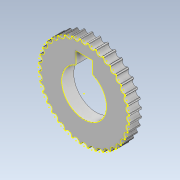
# Autodesk Inventor part: 2GT_36T
Saved by Autodesk Inventor 2022 (Build 260153000, 153)
## iProperties
Created: 2023-05-04
Part Number: 2GT_36T
Material: 一般
Document SubType Name: Modeling
Designer: Johnny Jou
Density: 1 g/cm^3
Appearance: 預設
Author: Johnny Jou
Autodesk Inventor part; units mm, degrees
ref_plane "YZ Plane" through (0, 0, 0) normal (1, 0, 0) x (0, 1, 0)
ref_plane "XZ Plane" through (0, 0, 0) normal (0, 1, 0) x (-1, 0, 0)
ref_plane "XY Plane" through (0, 0, 0) normal (0, 0, 1) x (1, 0, 0)
sketch "草圖1" plane through (0, 0, 0) normal (0, 0, 1) x (1, 0, 0)
  arc A0 (-2.6557, 10.7931) -> (-2.7562, 10.8607) centre (-2.7504, 10.7609) ccw
  arc A1 (-2.7562, 10.8607) -> (-3.0435, 10.7838) centre (0, 0) ccw
  arc A2 (-3.0435, 10.7838) -> (-3.0966, 10.675) centre (-2.9985, 10.6944) ccw
  arc A3 (-4.4896, 10.168) -> (-3.0966, 10.675) centre (-3.8323, 10.5293) ccw
  arc A4 (-4.4896, 10.168) -> (-4.6002, 10.2171) centre (-4.5772, 10.1198) ccw
  arc A5 (-4.6002, 10.2171) -> (-4.8698, 10.0914) centre (0, 0) ccw
  arc A6 (-4.8698, 10.0914) -> (-4.9033, 9.9751) centre (-4.81, 10.0113) ccw
  arc A7 (-6.187, 9.2339) -> (-4.9033, 9.9751) centre (-5.6025, 9.7038) ccw
  arc A8 (-6.187, 9.2339) -> (-6.3045, 9.2631) centre (-6.265, 9.1713) ccw
  arc A9 (-6.3045, 9.2631) -> (-6.5482, 9.0925) centre (0, 0) ccw
  arc A10 (-6.5482, 9.0925) -> (-6.5609, 8.9721) centre (-6.4754, 9.0239) ccw
  arc A11 (-7.6965, 8.0193) -> (-6.5609, 8.9721) centre (-7.2024, 8.5835) ccw
  arc A12 (-7.6965, 8.0193) -> (-7.8173, 8.0276) centre (-7.7624, 7.944) ccw
  arc A13 (-7.8173, 8.0276) -> (-8.0276, 7.8173) centre (0, 0) ccw
  arc A14 (-8.0276, 7.8173) -> (-8.0193, 7.6965) centre (-7.944, 7.7624) ccw
  arc A15 (-8.9721, 6.5609) -> (-8.0193, 7.6965) centre (-8.5835, 7.2024) ccw
  arc A16 (-8.9721, 6.5609) -> (-9.0925, 6.5482) centre (-9.0239, 6.4754) ccw
  arc A17 (-9.0925, 6.5482) -> (-9.2631, 6.3045) centre (0, 0) ccw
  arc A18 (-9.2631, 6.3045) -> (-9.2339, 6.187) centre (-9.1713, 6.265) ccw
  arc A19 (-9.9751, 4.9033) -> (-9.2339, 6.187) centre (-9.7038, 5.6025) ccw
  arc A20 (-9.9751, 4.9033) -> (-10.0914, 4.8698) centre (-10.0113, 4.81) ccw
  arc A21 (-10.0914, 4.8698) -> (-10.2171, 4.6002) centre (0, 0) ccw
  arc A22 (-10.2171, 4.6002) -> (-10.168, 4.4896) centre (-10.1198, 4.5772) ccw
  arc A23 (-10.675, 3.0966) -> (-10.168, 4.4896) centre (-10.5293, 3.8323) ccw
  arc A24 (-10.675, 3.0966) -> (-10.7838, 3.0435) centre (-10.6944, 2.9985) ccw
  arc A25 (-10.7838, 3.0435) -> (-10.8607, 2.7562) centre (0, 0) ccw
  arc A26 (-10.8607, 2.7562) -> (-10.7931, 2.6557) centre (-10.7609, 2.7504) ccw
  arc A27 (-11.0505, 1.1959) -> (-10.7931, 2.6557) centre (-11.0348, 1.9457) ccw
  arc A28 (-11.0505, 1.1959) -> (-11.1484, 1.1247) centre (-11.0526, 1.0959) ccw
  arc A29 (-11.1484, 1.1247) -> (-11.1743, 0.8283) centre (0, 0) ccw
  arc A30 (-11.1743, 0.8283) -> (-11.0903, 0.7412) centre (-11.075, 0.84) ccw
  arc A31 (-11.0903, -0.7412) -> (-11.0903, 0.7412) centre (-11.205, 0) ccw
  arc A32 (-11.0903, -0.7412) -> (-11.1743, -0.8283) centre (-11.075, -0.84) ccw
  arc A33 (-11.1743, -0.8283) -> (-11.1484, -1.1247) centre (0, 0) ccw
  arc A34 (-11.1484, -1.1247) -> (-11.0505, -1.1959) centre (-11.0526, -1.0959) ccw
  arc A35 (-10.7931, -2.6557) -> (-11.0505, -1.1959) centre (-11.0348, -1.9457) ccw
  arc A36 (-10.7931, -2.6557) -> (-10.8607, -2.7562) centre (-10.7609, -2.7504) ccw
  arc A37 (-10.8607, -2.7562) -> (-10.7838, -3.0435) centre (0, 0) ccw
  arc A38 (-10.7838, -3.0435) -> (-10.675, -3.0966) centre (-10.6944, -2.9985) ccw
  arc A39 (-10.168, -4.4896) -> (-10.675, -3.0966) centre (-10.5293, -3.8323) ccw
  arc A40 (-10.168, -4.4896) -> (-10.2171, -4.6002) centre (-10.1198, -4.5772) ccw
  arc A41 (-10.2171, -4.6002) -> (-10.0914, -4.8698) centre (0, 0) ccw
  arc A42 (-10.0914, -4.8698) -> (-9.9751, -4.9033) centre (-10.0113, -4.81) ccw
  arc A43 (-9.2339, -6.187) -> (-9.9751, -4.9033) centre (-9.7038, -5.6025) ccw
  arc A44 (-9.2339, -6.187) -> (-9.2631, -6.3045) centre (-9.1713, -6.265) ccw
  arc A45 (-9.2631, -6.3045) -> (-9.0925, -6.5482) centre (0, 0) ccw
  arc A46 (-9.0925, -6.5482) -> (-8.9721, -6.5609) centre (-9.0239, -6.4754) ccw
  arc A47 (-8.0193, -7.6965) -> (-8.9721, -6.5609) centre (-8.5835, -7.2024) ccw
  arc A48 (-8.0193, -7.6965) -> (-8.0276, -7.8173) centre (-7.944, -7.7624) ccw
  arc A49 (-8.0276, -7.8173) -> (-7.8173, -8.0276) centre (0, 0) ccw
  arc A50 (-7.8173, -8.0276) -> (-7.6965, -8.0193) centre (-7.7624, -7.944) ccw
  arc A51 (-6.5609, -8.9721) -> (-7.6965, -8.0193) centre (-7.2024, -8.5835) ccw
  arc A52 (-6.5609, -8.9721) -> (-6.5482, -9.0925) centre (-6.4754, -9.0239) ccw
  arc A53 (-6.5482, -9.0925) -> (-6.3045, -9.2631) centre (0, 0) ccw
  arc A54 (-6.3045, -9.2631) -> (-6.187, -9.2339) centre (-6.265, -9.1713) ccw
  arc A55 (-4.9033, -9.9751) -> (-6.187, -9.2339) centre (-5.6025, -9.7038) ccw
  arc A56 (-4.9033, -9.9751) -> (-4.8698, -10.0914) centre (-4.81, -10.0113) ccw
  arc A57 (-4.8698, -10.0914) -> (-4.6002, -10.2171) centre (0, 0) ccw
  arc A58 (-4.6002, -10.2171) -> (-4.4896, -10.168) centre (-4.5772, -10.1198) ccw
  arc A59 (-3.0966, -10.675) -> (-4.4896, -10.168) centre (-3.8323, -10.5293) ccw
  arc A60 (-3.0966, -10.675) -> (-3.0435, -10.7838) centre (-2.9985, -10.6944) ccw
  arc A61 (-3.0435, -10.7838) -> (-2.7562, -10.8607) centre (0, 0) ccw
  arc A62 (-2.7562, -10.8607) -> (-2.6557, -10.7931) centre (-2.7504, -10.7609) ccw
  arc A63 (-1.1959, -11.0505) -> (-2.6557, -10.7931) centre (-1.9457, -11.0348) ccw
  arc A64 (-1.1959, -11.0505) -> (-1.1247, -11.1484) centre (-1.0959, -11.0526) ccw
  arc A65 (-1.1247, -11.1484) -> (-0.8283, -11.1743) centre (0, 0) ccw
  arc A66 (-0.8283, -11.1743) -> (-0.7412, -11.0903) centre (-0.84, -11.075) ccw
  arc A67 (0.7412, -11.0903) -> (-0.7412, -11.0903) centre (0, -11.205) ccw
  arc A68 (0.7412, -11.0903) -> (0.8283, -11.1743) centre (0.84, -11.075) ccw
  arc A69 (0.8283, -11.1743) -> (1.1247, -11.1484) centre (0, 0) ccw
  arc A70 (1.1247, -11.1484) -> (1.1959, -11.0505) centre (1.0959, -11.0526) ccw
  arc A71 (2.6557, -10.7931) -> (1.1959, -11.0505) centre (1.9457, -11.0348) ccw
  arc A72 (2.6557, -10.7931) -> (2.7562, -10.8607) centre (2.7504, -10.7609) ccw
  arc A73 (2.7562, -10.8607) -> (3.0435, -10.7838) centre (0, 0) ccw
  arc A74 (3.0435, -10.7838) -> (3.0966, -10.675) centre (2.9985, -10.6944) ccw
  arc A75 (4.4896, -10.168) -> (3.0966, -10.675) centre (3.8323, -10.5293) ccw
  arc A76 (4.4896, -10.168) -> (4.6002, -10.2171) centre (4.5772, -10.1198) ccw
  arc A77 (4.6002, -10.2171) -> (4.8698, -10.0914) centre (0, 0) ccw
  arc A78 (4.8698, -10.0914) -> (4.9033, -9.9751) centre (4.81, -10.0113) ccw
  arc A79 (6.187, -9.2339) -> (4.9033, -9.9751) centre (5.6025, -9.7038) ccw
  arc A80 (6.187, -9.2339) -> (6.3045, -9.2631) centre (6.265, -9.1713) ccw
  arc A81 (6.3045, -9.2631) -> (6.5482, -9.0925) centre (0, 0) ccw
  arc A82 (6.5482, -9.0925) -> (6.5609, -8.9721) centre (6.4754, -9.0239) ccw
  arc A83 (7.6965, -8.0193) -> (6.5609, -8.9721) centre (7.2024, -8.5835) ccw
  arc A84 (7.6965, -8.0193) -> (7.8173, -8.0276) centre (7.7624, -7.944) ccw
  arc A85 (7.8173, -8.0276) -> (8.0276, -7.8173) centre (0, 0) ccw
  arc A86 (8.0276, -7.8173) -> (8.0193, -7.6965) centre (7.944, -7.7624) ccw
  arc A87 (8.9721, -6.5609) -> (8.0193, -7.6965) centre (8.5835, -7.2024) ccw
  arc A88 (8.9721, -6.5609) -> (9.0925, -6.5482) centre (9.0239, -6.4754) ccw
  arc A89 (9.0925, -6.5482) -> (9.2631, -6.3045) centre (0, 0) ccw
  arc A90 (9.2631, -6.3045) -> (9.2339, -6.187) centre (9.1713, -6.265) ccw
  arc A91 (9.9751, -4.9033) -> (9.2339, -6.187) centre (9.7038, -5.6025) ccw
  arc A92 (9.9751, -4.9033) -> (10.0914, -4.8698) centre (10.0113, -4.81) ccw
  arc A93 (10.0914, -4.8698) -> (10.2171, -4.6002) centre (0, 0) ccw
  arc A94 (10.2171, -4.6002) -> (10.168, -4.4896) centre (10.1198, -4.5772) ccw
  arc A95 (10.675, -3.0966) -> (10.168, -4.4896) centre (10.5293, -3.8323) ccw
  arc A96 (10.675, -3.0966) -> (10.7838, -3.0435) centre (10.6944, -2.9985) ccw
  arc A97 (10.7838, -3.0435) -> (10.8607, -2.7562) centre (0, 0) ccw
  arc A98 (10.8607, -2.7562) -> (10.7931, -2.6557) centre (10.7609, -2.7504) ccw
  arc A99 (11.0505, -1.1959) -> (10.7931, -2.6557) centre (11.0348, -1.9457) ccw
  arc A100 (11.0505, -1.1959) -> (11.1484, -1.1247) centre (11.0526, -1.0959) ccw
  arc A101 (11.1484, -1.1247) -> (11.1743, -0.8283) centre (0, 0) ccw
  arc A102 (11.1743, -0.8283) -> (11.0903, -0.7412) centre (11.075, -0.84) ccw
  arc A103 (11.0903, 0.7412) -> (11.0903, -0.7412) centre (11.205, 0) ccw
  arc A104 (11.0903, 0.7412) -> (11.1743, 0.8283) centre (11.075, 0.84) ccw
  arc A105 (11.1743, 0.8283) -> (11.1484, 1.1247) centre (0, 0) ccw
  arc A106 (11.1484, 1.1247) -> (11.0505, 1.1959) centre (11.0526, 1.0959) ccw
  arc A107 (10.7931, 2.6557) -> (11.0505, 1.1959) centre (11.0348, 1.9457) ccw
  arc A108 (10.7931, 2.6557) -> (10.8607, 2.7562) centre (10.7609, 2.7504) ccw
  arc A109 (10.8607, 2.7562) -> (10.7838, 3.0435) centre (0, 0) ccw
  arc A110 (10.7838, 3.0435) -> (10.675, 3.0966) centre (10.6944, 2.9985) ccw
  arc A111 (10.168, 4.4896) -> (10.675, 3.0966) centre (10.5293, 3.8323) ccw
  arc A112 (10.168, 4.4896) -> (10.2171, 4.6002) centre (10.1198, 4.5772) ccw
  arc A113 (10.2171, 4.6002) -> (10.0914, 4.8698) centre (0, 0) ccw
  arc A114 (10.0914, 4.8698) -> (9.9751, 4.9033) centre (10.0113, 4.81) ccw
  arc A115 (9.2339, 6.187) -> (9.9751, 4.9033) centre (9.7038, 5.6025) ccw
  arc A116 (9.2339, 6.187) -> (9.2631, 6.3045) centre (9.1713, 6.265) ccw
  arc A117 (9.2631, 6.3045) -> (9.0925, 6.5482) centre (0, 0) ccw
  arc A118 (9.0925, 6.5482) -> (8.9721, 6.5609) centre (9.0239, 6.4754) ccw
  arc A119 (8.0193, 7.6965) -> (8.9721, 6.5609) centre (8.5835, 7.2024) ccw
  arc A120 (8.0193, 7.6965) -> (8.0276, 7.8173) centre (7.944, 7.7624) ccw
  arc A121 (8.0276, 7.8173) -> (7.8173, 8.0276) centre (0, 0) ccw
  arc A122 (7.8173, 8.0276) -> (7.6965, 8.0193) centre (7.7624, 7.944) ccw
  arc A123 (6.5609, 8.9721) -> (7.6965, 8.0193) centre (7.2024, 8.5835) ccw
  arc A124 (6.5609, 8.9721) -> (6.5482, 9.0925) centre (6.4754, 9.0239) ccw
  arc A125 (6.5482, 9.0925) -> (6.3045, 9.2631) centre (0, 0) ccw
  arc A126 (6.3045, 9.2631) -> (6.187, 9.2339) centre (6.265, 9.1713) ccw
  arc A127 (4.9033, 9.9751) -> (6.187, 9.2339) centre (5.6025, 9.7038) ccw
  arc A128 (4.9033, 9.9751) -> (4.8698, 10.0914) centre (4.81, 10.0113) ccw
  arc A129 (4.8698, 10.0914) -> (4.6002, 10.2171) centre (0, 0) ccw
  arc A130 (4.6002, 10.2171) -> (4.4896, 10.168) centre (4.5772, 10.1198) ccw
  arc A131 (3.0966, 10.675) -> (4.4896, 10.168) centre (3.8323, 10.5293) ccw
  arc A132 (3.0966, 10.675) -> (3.0435, 10.7838) centre (2.9985, 10.6944) ccw
  arc A133 (3.0435, 10.7838) -> (2.7562, 10.8607) centre (0, 0) ccw
  arc A134 (2.7562, 10.8607) -> (2.6557, 10.7931) centre (2.7504, 10.7609) ccw
  arc A135 (1.1959, 11.0505) -> (2.6557, 10.7931) centre (1.9457, 11.0348) ccw
  arc A136 (1.1959, 11.0505) -> (1.1247, 11.1484) centre (1.0959, 11.0526) ccw
  arc A137 (1.1247, 11.1484) -> (0.8283, 11.1743) centre (0, 0) ccw
  arc A138 (0.8283, 11.1743) -> (0.7412, 11.0903) centre (0.84, 11.075) ccw
  arc A139 (-0.7412, 11.0903) -> (0.7412, 11.0903) centre (0, 11.205) ccw
  arc A140 (-0.7412, 11.0903) -> (-0.8283, 11.1743) centre (-0.84, 11.075) ccw
  arc A141 (-0.8283, 11.1743) -> (-1.1247, 11.1484) centre (0, 0) ccw
  arc A142 (-1.1247, 11.1484) -> (-1.1959, 11.0505) centre (-1.0959, 11.0526) ccw
  arc A143 (-2.6557, 10.7931) -> (-1.1959, 11.0505) centre (-1.9457, 11.0348) ccw
  circle A144 centre (0, 0) radius 5.5
  line L0 (-2, 8.1235) -> (2, 8.1235)
  line L1 (2, 8.1235) -> (2, 5.1235)
  line L2 (2, 5.1235) -> (-2, 5.1235)
  line L3 (-2, 5.1235) -> (-2, 8.1235)
  dimension "d0" = 11
  dimension "d1" = 4
  dimension "d2" = 3
  constraints: 290 point on circle, 145 centre point, 8 end point, 2 parallel, 1 coincident, 1 horizontal, 1 perpendicular, 396 other
  measures "d0" diameter of A144
  measures "d1" distance of L0.start L0.end
  measures "d2" distance of L0.end L1.end
extrude "擠出1" add sketch "草圖1" along normal blind 3
sketch "草圖2" plane through (0, 0, 3) normal (0, 0, 1) x (1, 0, 0)
  arc A0 (-2.7562, 10.8607) -> (-3.0435, 10.7838) centre (0, 0) ccw projected
  arc A1 (-3.0435, 10.7838) -> (-3.0966, 10.675) centre (-2.9985, 10.6944) ccw projected
  arc A2 (-4.4896, 10.168) -> (-3.0966, 10.675) centre (-3.8323, 10.5293) ccw projected
  arc A3 (-4.4896, 10.168) -> (-4.6002, 10.2171) centre (-4.5772, 10.1198) ccw projected
  arc A4 (-4.6002, 10.2171) -> (-4.8698, 10.0914) centre (0, 0) ccw projected
  arc A5 (-4.8698, 10.0914) -> (-4.9033, 9.9751) centre (-4.81, 10.0113) ccw projected
  arc A6 (-6.187, 9.2339) -> (-4.9033, 9.9751) centre (-5.6025, 9.7038) ccw projected
  arc A7 (-6.187, 9.2339) -> (-6.3045, 9.2631) centre (-6.265, 9.1713) ccw projected
  arc A8 (-6.3045, 9.2631) -> (-6.5482, 9.0925) centre (0, 0) ccw projected
  arc A9 (-6.5482, 9.0925) -> (-6.5609, 8.9721) centre (-6.4754, 9.0239) ccw projected
  arc A10 (-7.6965, 8.0193) -> (-6.5609, 8.9721) centre (-7.2024, 8.5835) ccw projected
  arc A11 (-7.6965, 8.0193) -> (-7.8173, 8.0276) centre (-7.7624, 7.944) ccw projected
  arc A12 (-7.8173, 8.0276) -> (-8.0276, 7.8173) centre (0, 0) ccw projected
  arc A13 (-8.0276, 7.8173) -> (-8.0193, 7.6965) centre (-7.944, 7.7624) ccw projected
  arc A14 (-8.9721, 6.5609) -> (-8.0193, 7.6965) centre (-8.5835, 7.2024) ccw projected
  arc A15 (-8.9721, 6.5609) -> (-9.0925, 6.5482) centre (-9.0239, 6.4754) ccw projected
  arc A16 (-9.0925, 6.5482) -> (-9.2631, 6.3045) centre (0, 0) ccw projected
  arc A17 (-9.2631, 6.3045) -> (-9.2339, 6.187) centre (-9.1713, 6.265) ccw projected
  arc A18 (-9.9751, 4.9033) -> (-9.2339, 6.187) centre (-9.7038, 5.6025) ccw projected
  arc A19 (-9.9751, 4.9033) -> (-10.0914, 4.8698) centre (-10.0113, 4.81) ccw projected
  arc A20 (-10.0914, 4.8698) -> (-10.2171, 4.6002) centre (0, 0) ccw projected
  arc A21 (-10.2171, 4.6002) -> (-10.168, 4.4896) centre (-10.1198, 4.5772) ccw projected
  arc A22 (-10.675, 3.0966) -> (-10.168, 4.4896) centre (-10.5293, 3.8323) ccw projected
  arc A23 (-10.675, 3.0966) -> (-10.7838, 3.0435) centre (-10.6944, 2.9985) ccw projected
  arc A24 (-10.7838, 3.0435) -> (-10.8607, 2.7562) centre (0, 0) ccw projected
  arc A25 (-10.8607, 2.7562) -> (-10.7931, 2.6557) centre (-10.7609, 2.7504) ccw projected
  arc A26 (-11.0505, 1.1959) -> (-10.7931, 2.6557) centre (-11.0348, 1.9457) ccw projected
  arc A27 (-11.0505, 1.1959) -> (-11.1484, 1.1247) centre (-11.0526, 1.0959) ccw projected
  arc A28 (-11.1484, 1.1247) -> (-11.1743, 0.8283) centre (0, 0) ccw projected
  arc A29 (-11.1743, 0.8283) -> (-11.0903, 0.7412) centre (-11.075, 0.84) ccw projected
  arc A30 (-11.0903, -0.7412) -> (-11.0903, 0.7412) centre (-11.205, 0) ccw projected
  arc A31 (-11.0903, -0.7412) -> (-11.1743, -0.8283) centre (-11.075, -0.84) ccw projected
  arc A32 (-11.1743, -0.8283) -> (-11.1484, -1.1247) centre (0, 0) ccw projected
  arc A33 (-11.1484, -1.1247) -> (-11.0505, -1.1959) centre (-11.0526, -1.0959) ccw projected
  arc A34 (-10.7931, -2.6557) -> (-11.0505, -1.1959) centre (-11.0348, -1.9457) ccw projected
  arc A35 (-10.7931, -2.6557) -> (-10.8607, -2.7562) centre (-10.7609, -2.7504) ccw projected
  arc A36 (-10.8607, -2.7562) -> (-10.7838, -3.0435) centre (0, 0) ccw projected
  arc A37 (-10.7838, -3.0435) -> (-10.675, -3.0966) centre (-10.6944, -2.9985) ccw projected
  arc A38 (-10.168, -4.4896) -> (-10.675, -3.0966) centre (-10.5293, -3.8323) ccw projected
  arc A39 (-10.168, -4.4896) -> (-10.2171, -4.6002) centre (-10.1198, -4.5772) ccw projected
  arc A40 (-10.2171, -4.6002) -> (-10.0914, -4.8698) centre (0, 0) ccw projected
  arc A41 (-10.0914, -4.8698) -> (-9.9751, -4.9033) centre (-10.0113, -4.81) ccw projected
  arc A42 (-9.2339, -6.187) -> (-9.9751, -4.9033) centre (-9.7038, -5.6025) ccw projected
  arc A43 (-9.2339, -6.187) -> (-9.2631, -6.3045) centre (-9.1713, -6.265) ccw projected
  arc A44 (-9.2631, -6.3045) -> (-9.0925, -6.5482) centre (0, 0) ccw projected
  arc A45 (-9.0925, -6.5482) -> (-8.9721, -6.5609) centre (-9.0239, -6.4754) ccw projected
  arc A46 (-8.0193, -7.6965) -> (-8.9721, -6.5609) centre (-8.5835, -7.2024) ccw projected
  arc A47 (-8.0193, -7.6965) -> (-8.0276, -7.8173) centre (-7.944, -7.7624) ccw projected
  arc A48 (-8.0276, -7.8173) -> (-7.8173, -8.0276) centre (0, 0) ccw projected
  arc A49 (-7.8173, -8.0276) -> (-7.6965, -8.0193) centre (-7.7624, -7.944) ccw projected
  arc A50 (-6.5609, -8.9721) -> (-7.6965, -8.0193) centre (-7.2024, -8.5835) ccw projected
  arc A51 (-6.5609, -8.9721) -> (-6.5482, -9.0925) centre (-6.4754, -9.0239) ccw projected
  arc A52 (-6.5482, -9.0925) -> (-6.3045, -9.2631) centre (0, 0) ccw projected
  arc A53 (-6.3045, -9.2631) -> (-6.187, -9.2339) centre (-6.265, -9.1713) ccw projected
  arc A54 (-4.9033, -9.9751) -> (-6.187, -9.2339) centre (-5.6025, -9.7038) ccw projected
  arc A55 (-4.9033, -9.9751) -> (-4.8698, -10.0914) centre (-4.81, -10.0113) ccw projected
  arc A56 (-4.8698, -10.0914) -> (-4.6002, -10.2171) centre (0, 0) ccw projected
  arc A57 (-4.6002, -10.2171) -> (-4.4896, -10.168) centre (-4.5772, -10.1198) ccw projected
  arc A58 (-3.0966, -10.675) -> (-4.4896, -10.168) centre (-3.8323, -10.5293) ccw projected
  arc A59 (-3.0966, -10.675) -> (-3.0435, -10.7838) centre (-2.9985, -10.6944) ccw projected
  arc A60 (-3.0435, -10.7838) -> (-2.7562, -10.8607) centre (0, 0) ccw projected
  arc A61 (-2.7562, -10.8607) -> (-2.6557, -10.7931) centre (-2.7504, -10.7609) ccw projected
  arc A62 (-1.1959, -11.0505) -> (-2.6557, -10.7931) centre (-1.9457, -11.0348) ccw projected
  arc A63 (-1.1959, -11.0505) -> (-1.1247, -11.1484) centre (-1.0959, -11.0526) ccw projected
  arc A64 (-1.1247, -11.1484) -> (-0.8283, -11.1743) centre (0, 0) ccw projected
  arc A65 (-0.8283, -11.1743) -> (-0.7412, -11.0903) centre (-0.84, -11.075) ccw projected
  arc A66 (0.7412, -11.0903) -> (-0.7412, -11.0903) centre (0, -11.205) ccw projected
  arc A67 (0.7412, -11.0903) -> (0.8283, -11.1743) centre (0.84, -11.075) ccw projected
  arc A68 (0.8283, -11.1743) -> (1.1247, -11.1484) centre (0, 0) ccw projected
  arc A69 (1.1247, -11.1484) -> (1.1959, -11.0505) centre (1.0959, -11.0526) ccw projected
  arc A70 (2.6557, -10.7931) -> (1.1959, -11.0505) centre (1.9457, -11.0348) ccw projected
  arc A71 (2.6557, -10.7931) -> (2.7562, -10.8607) centre (2.7504, -10.7609) ccw projected
  arc A72 (2.7562, -10.8607) -> (3.0435, -10.7838) centre (0, 0) ccw projected
  arc A73 (3.0435, -10.7838) -> (3.0966, -10.675) centre (2.9985, -10.6944) ccw projected
  arc A74 (4.4896, -10.168) -> (3.0966, -10.675) centre (3.8323, -10.5293) ccw projected
  arc A75 (4.4896, -10.168) -> (4.6002, -10.2171) centre (4.5772, -10.1198) ccw projected
  arc A76 (4.6002, -10.2171) -> (4.8698, -10.0914) centre (0, 0) ccw projected
  arc A77 (4.8698, -10.0914) -> (4.9033, -9.9751) centre (4.81, -10.0113) ccw projected
  arc A78 (6.187, -9.2339) -> (4.9033, -9.9751) centre (5.6025, -9.7038) ccw projected
  arc A79 (6.187, -9.2339) -> (6.3045, -9.2631) centre (6.265, -9.1713) ccw projected
  arc A80 (6.3045, -9.2631) -> (6.5482, -9.0925) centre (0, 0) ccw projected
  arc A81 (6.5482, -9.0925) -> (6.5609, -8.9721) centre (6.4754, -9.0239) ccw projected
  arc A82 (7.6965, -8.0193) -> (6.5609, -8.9721) centre (7.2024, -8.5835) ccw projected
  arc A83 (7.6965, -8.0193) -> (7.8173, -8.0276) centre (7.7624, -7.944) ccw projected
  arc A84 (7.8173, -8.0276) -> (8.0276, -7.8173) centre (0, 0) ccw projected
  arc A85 (8.0276, -7.8173) -> (8.0193, -7.6965) centre (7.944, -7.7624) ccw projected
  arc A86 (8.9721, -6.5609) -> (8.0193, -7.6965) centre (8.5835, -7.2024) ccw projected
  arc A87 (8.9721, -6.5609) -> (9.0925, -6.5482) centre (9.0239, -6.4754) ccw projected
  arc A88 (9.0925, -6.5482) -> (9.2631, -6.3045) centre (0, 0) ccw projected
  arc A89 (9.2631, -6.3045) -> (9.2339, -6.187) centre (9.1713, -6.265) ccw projected
  arc A90 (9.9751, -4.9033) -> (9.2339, -6.187) centre (9.7038, -5.6025) ccw projected
  arc A91 (9.9751, -4.9033) -> (10.0914, -4.8698) centre (10.0113, -4.81) ccw projected
  arc A92 (10.0914, -4.8698) -> (10.2171, -4.6002) centre (0, 0) ccw projected
  arc A93 (10.2171, -4.6002) -> (10.168, -4.4896) centre (10.1198, -4.5772) ccw projected
  arc A94 (10.675, -3.0966) -> (10.168, -4.4896) centre (10.5293, -3.8323) ccw projected
  arc A95 (10.675, -3.0966) -> (10.7838, -3.0435) centre (10.6944, -2.9985) ccw projected
  arc A96 (10.7838, -3.0435) -> (10.8607, -2.7562) centre (0, 0) ccw projected
  arc A97 (10.8607, -2.7562) -> (10.7931, -2.6557) centre (10.7609, -2.7504) ccw projected
  arc A98 (11.0505, -1.1959) -> (10.7931, -2.6557) centre (11.0348, -1.9457) ccw projected
  arc A99 (11.0505, -1.1959) -> (11.1484, -1.1247) centre (11.0526, -1.0959) ccw projected
  arc A100 (11.1484, -1.1247) -> (11.1743, -0.8283) centre (0, 0) ccw projected
  arc A101 (11.1743, -0.8283) -> (11.0903, -0.7412) centre (11.075, -0.84) ccw projected
  arc A102 (11.0903, 0.7412) -> (11.0903, -0.7412) centre (11.205, 0) ccw projected
  arc A103 (11.0903, 0.7412) -> (11.1743, 0.8283) centre (11.075, 0.84) ccw projected
  arc A104 (11.1743, 0.8283) -> (11.1484, 1.1247) centre (0, 0) ccw projected
  arc A105 (11.1484, 1.1247) -> (11.0505, 1.1959) centre (11.0526, 1.0959) ccw projected
  arc A106 (10.7931, 2.6557) -> (11.0505, 1.1959) centre (11.0348, 1.9457) ccw projected
  arc A107 (10.7931, 2.6557) -> (10.8607, 2.7562) centre (10.7609, 2.7504) ccw projected
  arc A108 (10.8607, 2.7562) -> (10.7838, 3.0435) centre (0, 0) ccw projected
  arc A109 (10.7838, 3.0435) -> (10.675, 3.0966) centre (10.6944, 2.9985) ccw projected
  arc A110 (10.168, 4.4896) -> (10.675, 3.0966) centre (10.5293, 3.8323) ccw projected
  arc A111 (10.168, 4.4896) -> (10.2171, 4.6002) centre (10.1198, 4.5772) ccw projected
  arc A112 (10.2171, 4.6002) -> (10.0914, 4.8698) centre (0, 0) ccw projected
  arc A113 (10.0914, 4.8698) -> (9.9751, 4.9033) centre (10.0113, 4.81) ccw projected
  arc A114 (9.2339, 6.187) -> (9.9751, 4.9033) centre (9.7038, 5.6025) ccw projected
  arc A115 (9.2339, 6.187) -> (9.2631, 6.3045) centre (9.1713, 6.265) ccw projected
  arc A116 (9.2631, 6.3045) -> (9.0925, 6.5482) centre (0, 0) ccw projected
  arc A117 (9.0925, 6.5482) -> (8.9721, 6.5609) centre (9.0239, 6.4754) ccw projected
  arc A118 (8.0193, 7.6965) -> (8.9721, 6.5609) centre (8.5835, 7.2024) ccw projected
  arc A119 (8.0193, 7.6965) -> (8.0276, 7.8173) centre (7.944, 7.7624) ccw projected
  arc A120 (8.0276, 7.8173) -> (7.8173, 8.0276) centre (0, 0) ccw projected
  arc A121 (7.8173, 8.0276) -> (7.6965, 8.0193) centre (7.7624, 7.944) ccw projected
  arc A122 (6.5609, 8.9721) -> (7.6965, 8.0193) centre (7.2024, 8.5835) ccw projected
  arc A123 (6.5609, 8.9721) -> (6.5482, 9.0925) centre (6.4754, 9.0239) ccw projected
  arc A124 (6.5482, 9.0925) -> (6.3045, 9.2631) centre (0, 0) ccw projected
  arc A125 (6.3045, 9.2631) -> (6.187, 9.2339) centre (6.265, 9.1713) ccw projected
  arc A126 (4.9033, 9.9751) -> (6.187, 9.2339) centre (5.6025, 9.7038) ccw projected
  arc A127 (4.9033, 9.9751) -> (4.8698, 10.0914) centre (4.81, 10.0113) ccw projected
  arc A128 (4.8698, 10.0914) -> (4.6002, 10.2171) centre (0, 0) ccw projected
  arc A129 (4.6002, 10.2171) -> (4.4896, 10.168) centre (4.5772, 10.1198) ccw projected
  arc A130 (3.0966, 10.675) -> (4.4896, 10.168) centre (3.8323, 10.5293) ccw projected
  arc A131 (3.0966, 10.675) -> (3.0435, 10.7838) centre (2.9985, 10.6944) ccw projected
  arc A132 (3.0435, 10.7838) -> (2.7562, 10.8607) centre (0, 0) ccw projected
  arc A133 (2.7562, 10.8607) -> (2.6557, 10.7931) centre (2.7504, 10.7609) ccw projected
  arc A134 (1.1959, 11.0505) -> (2.6557, 10.7931) centre (1.9457, 11.0348) ccw projected
  arc A135 (1.1959, 11.0505) -> (1.1247, 11.1484) centre (1.0959, 11.0526) ccw projected
  arc A136 (1.1247, 11.1484) -> (0.8283, 11.1743) centre (0, 0) ccw projected
  arc A137 (0.8283, 11.1743) -> (0.7412, 11.0903) centre (0.84, 11.075) ccw projected
  arc A138 (-0.7412, 11.0903) -> (0.7412, 11.0903) centre (0, 11.205) ccw projected
  arc A139 (-0.7412, 11.0903) -> (-0.8283, 11.1743) centre (-0.84, 11.075) ccw projected
  arc A140 (-0.8283, 11.1743) -> (-1.1247, 11.1484) centre (0, 0) ccw projected
  arc A141 (-1.1247, 11.1484) -> (-1.1959, 11.0505) centre (-1.0959, 11.0526) ccw projected
  arc A142 (-2.6557, 10.7931) -> (-1.1959, 11.0505) centre (-1.9457, 11.0348) ccw projected
  arc A143 (-2.6557, 10.7931) -> (-2.7562, 10.8607) centre (-2.7504, 10.7609) ccw projected
  line L0 (-2, 8.1235) -> (2, 8.1235) projected
  line L1 (2, 8.1235) -> (2, 5.1235) projected
  arc A144 (-2, 5.1235) -> (2, 5.1235) centre (0, 0) ccw projected
  line L2 (-2, 5.1235) -> (-2, 8.1235) projected
